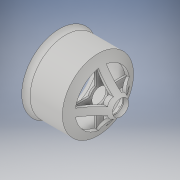
# Autodesk Inventor part: ducted fan barrel
Saved by Autodesk Inventor 2019 (Build 230136000, 136)
## iProperties
Created: 2020-03-27
Part Number: ducted fan barrel
Material: Generic
Document SubType Name: Modeling
Designer: q
Density: 1 g/cm^3
Appearance: Default
Author: q
Autodesk Inventor part; units mm, degrees
ref_plane "YZ Plane" through (0, 0, 0) normal (1, 0, 0) x (0, 1, 0)
ref_plane "XZ Plane" through (0, 0, 0) normal (0, 1, 0) x (-1, 0, 0)
ref_plane "XY Plane" through (0, 0, 0) normal (0, 0, 1) x (1, 0, 0)
sketch "Sketch1" plane through (0, 0, 0) normal (0, 1, 0) x (-1, 0, 0)
  line L0 (0, 0) -> (0, -501)
  line L1 (0, 0) -> (45.73955, 0)
  line L2 (0, -551) -> (500, -551)
  line L3 (0, -501) -> (500.813716, -501)
  arc A0 (597.473287, -583.490518) -> (500.813716, -501) centre (500.813716, -598.87645) ccw
  arc A1 (597.473287, -583.490518) -> (500, -551) centre (521.039168, -650.339163) ccw
  arc A2 (0, -551) -> (-500, -40.925823) centre (-905.168086, -938.191155) ccw
  line L4 (-500, 0) -> (-500, -40.925823)
  line L5 (0, 0) -> (-30, 0)
  line L6 (-30, 0) -> (-30, -417.068105)
  arc A3 (-30, -417.068105) -> (-500, 0) centre (-822.460207, -836.743915) ccw
  line L7 (0, 0) -> (-30, 0)
  dimension "d0" = 501
  dimension "d1" = 50
  dimension "d2" = 500
  dimension "d3" = 500
  dimension "d4" = 30
  constraints: 16 end point, 8 point on circle, 4 centre point, 2 horizontal, 2 vertical, 1 collinear, 1 perpendicular, 1 tangent
  measures "d0" distance of L0.start L0.end
  measures "d1" distance of L0.end L2.start
  measures "d2" distance of L2.start L2.end
  measures "d3" distance of L0.start L4.start
  measures "d4" distance of L0.start L5.end
sketch "Sketch1 outline for Revolution1" plane through (0, 0, 0) normal (0, 1, 0) x (-1, 0, 0)
  line L0 (0, -501) -> (0, 0)
  line L1 (500.813716, -501) -> (0, -501)
  arc A0 (597.473287, -583.490518) -> (500.813716, -501) centre (500.813716, -598.87645) ccw
  arc A1 (500, -551) -> (597.473287, -583.490518) centre (521.039168, -650.339163) cw
  line L2 (0, -551) -> (500, -551)
  arc A2 (-500, -40.925823) -> (0, -551) centre (-905.168086, -938.191155) cw
  line L3 (-500, 0) -> (-500, -40.925823)
  arc A3 (-30, -417.068105) -> (-500, 0) centre (-822.460207, -836.743915) ccw
  line L4 (-30, 0) -> (-30, -417.068105)
  line L5 (0, 0) -> (-30, 0)
revolve "Revolution1" add sketch "Sketch1 outline for Revolution1" angle 360 about axis through (0, 0, 0) along (-1, 0, 0)
sketch "Sketch2" plane through (0, 0, 0) normal (-1, 0, 0) x (0, 0, 1)
  circle A0 centre (0, 0) radius 40.925823
  circle A1 centre (0, 0) radius 125
  circle A2 centre (0, 0) radius 450
  circle A3 centre (0, 0) radius 417.068105
  arc A4 (60, -417.068105) -> (417.068105, -60) centre (-16.008639, 16.008639) ccw
  arc A5 (60, -149.658561) -> (149.658561, -60) centre (33.046302, -33.046302) ccw
  line L0 (149.658561, -60) -> (417.068105, -60)
  line L1 (60, -149.658561) -> (60, -417.068105)
  line L2 (60, 149.658561) -> (60, 417.068105)
  arc A6 (149.658561, 60) -> (60, 149.658561) centre (33.046302, 33.046302) ccw
  line L3 (149.658561, 60) -> (417.068105, 60)
  arc A7 (417.068105, 60) -> (60, 417.068105) centre (-16.008639, -16.008639) ccw
  line L4 (-149.658561, 60) -> (-417.068105, 60)
  arc A8 (-60, 149.658561) -> (-149.658561, 60) centre (-33.046302, 33.046302) ccw
  line L5 (-60, 149.658561) -> (-60, 417.068105)
  arc A9 (-60, 417.068105) -> (-417.068105, 60) centre (16.008639, -16.008639) ccw
  line L6 (-60, -149.658561) -> (-60, -417.068105)
  arc A10 (-149.658561, -60) -> (-60, -149.658561) centre (-33.046302, -33.046302) ccw
  line L7 (-149.658561, -60) -> (-417.068105, -60)
  arc A11 (-417.068105, -60) -> (-60, -417.068105) centre (16.008639, 16.008639) ccw
  dimension "d6" = 250
  dimension "d7" = 900
  dimension "d15" = 360
  constraints: 16 end point, 16 point on circle, 10 centre point, 2 coincident, 1 horizontal, 1 perpendicular, 41 other
  measures "d6" diameter of A1
  measures "d7" diameter of A2
sketch "Sketch2 outline for Extrusion1" plane through (0, 0, 0) normal (-1, 0, 0) x (0, 0, 1)
  line L0 (60, -149.658561) -> (60, -417.068105)
  arc A0 (149.658561, -60) -> (60, -149.658561) centre (33.046302, -33.046302) cw
  line L1 (417.068105, -60) -> (149.658561, -60)
  arc A1 (60, -417.068105) -> (417.068105, -60) centre (-16.008639, 16.008639) ccw
  line L2 (60, 417.068105) -> (60, 149.658561)
  arc A2 (417.068105, 60) -> (60, 417.068105) centre (-16.008639, -16.008639) ccw
  line L3 (149.658561, 60) -> (417.068105, 60)
  arc A3 (60, 149.658561) -> (149.658561, 60) centre (33.046302, 33.046302) cw
  line L4 (-417.068105, 60) -> (-149.658561, 60)
  arc A4 (-60, 417.068105) -> (-417.068105, 60) centre (16.008639, -16.008639) ccw
  line L5 (-60, 149.658561) -> (-60, 417.068105)
  arc A5 (-149.658561, 60) -> (-60, 149.658561) centre (-33.046302, 33.046302) cw
  line L6 (-60, -417.068105) -> (-60, -149.658561)
  arc A6 (-417.068105, -60) -> (-60, -417.068105) centre (16.008639, 16.008639) ccw
  line L7 (-149.658561, -60) -> (-417.068105, -60)
  arc A7 (-60, -149.658561) -> (-149.658561, -60) centre (-33.046302, -33.046302) cw
  circle A8 centre (0, 0) radius 125
  circle A9 centre (0, 0) radius 40.925823
extrude "Extrusion1" cut sketch "Sketch2 outline for Extrusion1" against normal blind 1000
sketch "Sketch3" plane through (0, 0, 0) normal (-1, 0, 0) x (0, 0, 1)
  circle A0 centre (0, 0) radius 46.553893
  constraints: 1 centre point, 1 coincident
sketch "Sketch3 outline for Extrusion2" plane through (0, 0, 0) normal (-1, 0, 0) x (0, 0, 1)
  circle A0 centre (0, 0) radius 46.553893
extrude "Extrusion2" cut sketch "Sketch3 outline for Extrusion2" against normal blind 1000
body "Solid1"
